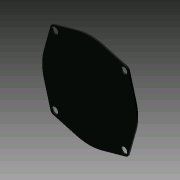
# Autodesk Inventor part: Back Plate 2 1764
Saved by Autodesk Inventor 2011 (Build 150239000, 239)
## iProperties
Created: 2010-02-23
Part Number: Back Plate 2 1764
Document SubType Name: Modeling
Designer: jgehrig
Density: 1 g/cm^3
Author: jgehrig
Autodesk Inventor part; units mm, degrees
ref_plane "YZ Plane" through (0, 0, 0) normal (1, 0, 0) x (0, 1, 0)
ref_plane "XZ Plane" through (0, 0, 0) normal (0, 1, 0) x (-1, 0, 0)
ref_plane "XY Plane" through (0, 0, 0) normal (0, 0, 1) x (1, 0, 0)
sketch "Sketch1" plane through (0, 0, 0) normal (0, 0, 1) x (1, 0, 0)
  circle A0 centre (31.115, 31.115) radius 2.8575
  line L0 (35.0538, 32.8409) -> (41.0029, 11.3509)
  arc A1 (35.0538, 32.8409) -> (32.8409, 35.0538) centre (31.9938, 31.9938) ccw
  line L1 (11.3509, 41.0029) -> (32.8409, 35.0538)
  arc A2 (41.0029, -11.3509) -> (41.0029, 11.3509) centre (0, 0) ccw
  line L2 (41.0029, -11.3509) -> (35.0538, -32.8409)
  line L3 (32.8409, -35.0538) -> (11.3509, -41.0029)
  arc A3 (32.8409, -35.0538) -> (35.0538, -32.8409) centre (31.9938, -31.9938) ccw
  arc A4 (-11.3509, -41.0029) -> (11.3509, -41.0029) centre (0, 0) ccw
  line L4 (-11.3509, -41.0029) -> (-32.8409, -35.0538)
  arc A5 (-35.0538, -32.8409) -> (-32.8409, -35.0538) centre (-31.9938, -31.9938) ccw
  line L5 (-35.0538, -32.8409) -> (-41.0029, -11.3509)
  arc A6 (-41.0029, 11.3509) -> (-41.0029, -11.3509) centre (0, 0) ccw
  line L6 (-41.0029, 11.3509) -> (-35.0538, 32.8409)
  arc A7 (-32.8409, 35.0538) -> (-35.0538, 32.8409) centre (-31.9938, 31.9938) ccw
  line L7 (-32.8409, 35.0538) -> (-11.3509, 41.0029)
  circle A8 centre (-31.115, 31.115) radius 2.8575
  circle A9 centre (-31.115, 31.115) radius 1.5875
  circle A10 centre (31.115, 31.115) radius 1.5875
  circle A11 centre (31.115, -31.115) radius 2.8575
  circle A12 centre (31.115, -31.115) radius 1.5875
  circle A13 centre (-31.115, -31.115) radius 2.8575
  circle A14 centre (-31.115, -31.115) radius 1.5875
  arc A15 (11.3509, 41.0029) -> (-11.3509, 41.0029) centre (0, 0) ccw
  point P0 (0, 0)
  constraints: 16 centre point, 16 end point, 16 point on circle
extrude "Extrusion1" add sketch "Sketch1" along normal blind 1.27 contours L0 A2 L2 A3 L3 A4 L4 A5 L5 A6 L6 A7 L7 A15 L1 A1
body "Solid1"
